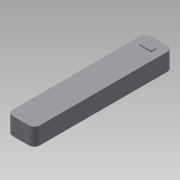
# Autodesk Inventor part: power strip
Saved by Autodesk Inventor 2015 (Build 190159000, 159)
## iProperties
Created: 2015-05-22
Part Number: power strip
Material: Generic
Document SubType Name: Modeling
Designer: Joe Sheldon
Density: 1 g/cm^3
Appearance: Default
Author: Joe Sheldon
Autodesk Inventor part; units mm, degrees
ref_plane "YZ Plane" through (0, 0, 0) normal (1, 0, 0) x (0, 1, 0)
ref_plane "XZ Plane" through (0, 0, 0) normal (0, 1, 0) x (-1, 0, 0)
ref_plane "XY Plane" through (0, 0, 0) normal (0, 0, 1) x (1, 0, 0)
sketch "Sketch1" plane through (0, 0, 0) normal (0, 1, 0) x (-1, 0, 0)
  line L0 (0, 0) -> (69.85, 0)
  line L1 (69.85, 0) -> (69.85, -355.6)
  line L2 (69.85, -355.6) -> (0, -355.6)
  line L3 (0, -355.6) -> (0, 0)
  dimension "d0" = 69.85
  dimension "d1" = 355.6
  constraints: 8 end point, 2 parallel, 1 horizontal, 1 perpendicular
  measures "d0" distance of L1.end L2.end
  measures "d1" distance of L0.end L1.end
extrude "Extrusion1" add sketch "Sketch1" along normal blind 44.45
fillet "Fillet1" radius 14.2875 4 edges at (0, 22.225, 0) (-69.85, 22.225, 0) (0, 22.225, -355.6) (-69.85, 22.225, -355.6)
sketch "Sketch3" plane through (0, 44.45, 0) normal (0, 1, 0) x (1, 0, 0)
  arc A0 (-55.5625, 355.6) -> (-69.85, 341.3125) centre (-55.5625, 341.3125) ccw projected
  line L0 (-69.85, 341.3125) -> (-69.85, 14.2875) projected
  arc A1 (-69.85, 14.2875) -> (-55.5625, 0) centre (-55.5625, 14.2875) ccw projected
  line L1 (-55.5625, 0) -> (-14.2875, 0) projected
  arc A2 (-14.2875, 0) -> (0, 14.2875) centre (-14.2875, 14.2875) ccw projected
  line L2 (0, 14.2875) -> (0, 341.3125) projected
  arc A3 (0, 341.3125) -> (-14.2875, 355.6) centre (-14.2875, 341.3125) ccw projected
  line L3 (-14.2875, 355.6) -> (-55.5625, 355.6) projected
  line L4 (-19.685, 333.0203) -> (-50.165, 333.0203)
  line L5 (-50.165, 333.0203) -> (-50.165, 319.6698)
  line L6 (-50.165, 319.6698) -> (-19.685, 319.6698)
  line L7 (-19.685, 319.6698) -> (-19.685, 333.0203)
  line L8 (-19.685, 333.0203) -> (-50.165, 319.6698) construction
  line L9 (-50.165, 333.0203) -> (-19.685, 319.6698) construction
  point P0 (0, 0)
  point P1 (-34.925, 326.345)
  constraints: 12 end point, 2 midpoint, 2 parallel, 1 horizontal, 1 perpendicular
extrude "Extrusion3" add sketch "Sketch3" along normal blind 3.175 contours L7 L6 L5 L4
body "Solid1"
